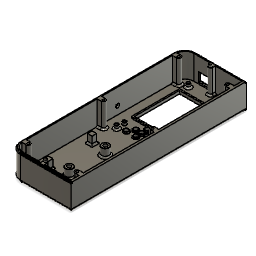
Front_panel_rev_C+ (Autodesk Fusion 360 design; units mm, degrees)
Autodesk Fusion 360 part; units mm, degrees
sketch "Sketch1" plane through (0, 0, 0) normal (0, 1, 0) x (1, 0, 0)
  line L0 (-20, 50) -> (62, 50)
  line L1 (62, 50) -> (62, -183)
  line L2 (62, -183) -> (-20, -183)
  line L3 (-20, -183) -> (-20, 50)
  dimension "d1" = 233
  dimension "d2" = 82
  dimension "d62" = 0
  dimension "d63" = 0
  dimension "d64" = 0
  dimension "d65" = 0
  constraint horizontal L0
  constraint vertical L1
  constraint horizontal L2
  constraint vertical L3
  measures "d1" distance of L0.start L2.end
  measures "d2" distance of L0.start L0.end
extrude "Extrude1" add sketch "Sketch1" along normal blind 35
fillet "Fillet1" radius 15 2 edges at (-20, 17.5, -50) (-20, 17.5, 183)
shell "Shell1" thickness 3 removed faces 1 at (34.6667, 35, 32.6667)
sketch "Sketch2" plane through (0, 35, 0) normal (0, 1, 0) x (-1, 0, 0)
  arc A0 (5, -47) -> (17, -35) centre (5, -35) ccw
  line L0 (5, -47) -> (-59, -47)
  line L1 (-59, -47) -> (-59, 180)
  line L2 (-59, 180) -> (5, 180)
  arc A1 (17, 168) -> (5, 180) centre (5, 168) ccw
  line L3 (17, 168) -> (17, -35)
  arc A2 (20, 168) -> (5, 183) centre (5, 168) ccw
  line L4 (5, 183) -> (-62, 183)
  line L5 (-62, 183) -> (-62, -50)
  line L6 (-62, -50) -> (5, -50)
  arc A3 (5, -50) -> (20, -35) centre (5, -35) ccw
  line L7 (20, -35) -> (20, 168)
  line L8 (-62, -48.5) -> (5, -48.5)
  arc A4 (5, -48.5) -> (18.5, -35) centre (5, -35) ccw
  line L9 (18.5, -35) -> (18.5, 168)
  arc A5 (18.5, 168) -> (5, 181.5) centre (5, 168) ccw
  line L10 (5, 181.5) -> (-62, 181.5)
  dimension "d7" = 1.5
extrude "Extrude2" cut sketch "Sketch2" against normal blind 1.6 contours A2 L4 L5 L6 A3 L7 L8 A4 L9 A5 L10
sketch "Sketch3" plane through (0, 3, 0) normal (0, 1, 0) x (-1, 0, 0)
  arc A0 (17, 168) -> (5, 180) centre (5, 168) ccw
  line L0 (5, 180) -> (-59, 180)
  line L1 (-59, 180) -> (-59, -47)
  line L2 (-59, -47) -> (5, -47)
  arc A1 (5, -47) -> (17, -35) centre (5, -35) ccw
  line L3 (17, -35) -> (17, 168)
  circle A2 centre (-21, 176) radius 2.5
  line L4 (-62, 181.5) -> (-62, -48.5)
  line L5 (-62, 183) -> (5, 183)
  circle A3 centre (-21, -43) radius 2.5
  line L6 (5, -50) -> (-62, -50)
  line L7 (20, 168) -> (20, -35) construction
  line L8 (-62, 66.5) -> (20, 66.5) construction
  circle A4 centre (11.5, 66.5) radius 3
  circle A5 centre (-53.5, 66.5) radius 3
  line L9 (-21, 230) -> (-21, -74.0636) construction
  line L10 (11.5, 191.1088) -> (11.5, -90) construction
  line L11 (-53.5, -65.1601) -> (-53.5, 224.5392) construction
  circle A6 centre (11.5, 166.5) radius 3
  circle A7 centre (-53.5, 166.5) radius 3
  circle A8 centre (11.5, -33.5) radius 3
  circle A9 centre (-53.5, -33.5) radius 3
  line L12 (-53.5, 169.5) -> (-59, 169.5)
  line L13 (-53.5, 163.5) -> (-59, 163.5)
  line L14 (11.5, 169.5) -> (16.9059, 169.5)
  line L15 (11.5, 163.5) -> (17, 163.5)
  line L16 (11.5, 63.5) -> (17, 63.5)
  line L17 (11.5, 69.5) -> (17, 69.5)
  line L18 (-53.5, 63.5) -> (-59, 63.5)
  line L19 (-53.5, 69.5) -> (-59, 69.5)
  line L20 (11.5, -36.5) -> (16.9059, -36.5)
  line L21 (11.5, -30.5) -> (17, -30.5)
  line L22 (-18.5, -43) -> (-18.5, -47)
  line L23 (-23.5, -43) -> (-23.5, -47)
  line L24 (-23.5, 176) -> (-23.5, 180)
  line L25 (-18.5, 176) -> (-18.5, 180)
  line L26 (-53.5, -30.5) -> (-59, -30.5)
  line L27 (-53.5, -36.5) -> (-59, -36.5)
  line L28 (-46.4, 61) -> (4.4, 61)
  line L29 (4.4, 61) -> (4.4, -39)
  line L30 (4.4, -39) -> (-46.4, -39)
  line L31 (-46.4, -39) -> (-46.4, 61)
  line L32 (-46.4, 61) -> (4.4, -39) construction
  line L33 (4.4, 61) -> (-46.4, -39) construction
  line L34 (-43.86, 58.625) -> (1.86, 58.625)
  line L35 (1.86, 58.625) -> (1.86, -36.625)
  line L36 (1.86, -36.625) -> (-43.86, -36.625)
  line L37 (-43.86, -36.625) -> (-43.86, 58.625)
  line L38 (-43.86, 58.625) -> (1.86, -36.625) construction
  line L39 (1.86, 58.625) -> (-43.86, -36.625) construction
  circle A10 centre (1.86, -36.625) radius 1.5
  circle A11 centre (-43.86, -36.625) radius 2.5
  circle A12 centre (-43.86, -36.625) radius 1.5
  circle A13 centre (1.86, -36.625) radius 2.5
  circle A14 centre (1.86, 58.625) radius 2.5
  circle A15 centre (1.86, 58.625) radius 1.5
  circle A16 centre (-43.86, 58.625) radius 2.5
  circle A17 centre (-43.86, 58.625) radius 1.5
  line L40 (-43.5, 149.6675) -> (1.5, 149.6675)
  line L41 (1.5, 149.6675) -> (1.5, 91.6675)
  line L42 (1.5, 91.6675) -> (-43.5, 91.6675)
  line L43 (-43.5, 91.6675) -> (-43.5, 149.6675)
  line L44 (-43.5, 149.6675) -> (1.5, 91.6675) construction
  line L45 (1.5, 149.6675) -> (-43.5, 91.6675) construction
  circle A18 centre (-21, 144.6675) radius 2.5
  circle A19 centre (-21, 96.6675) radius 2.5
  circle A20 centre (-21, 96.6675) radius 5
  circle A21 centre (-21, 144.6675) radius 5
  line L46 (-1.5, 94.6675) -> (4.5, 94.6675)
  line L47 (4.5, 94.6675) -> (4.5, 88.6675)
  line L48 (4.5, 88.6675) -> (-1.5, 88.6675)
  line L49 (-1.5, 88.6675) -> (-1.5, 94.6675)
  line L50 (-1.5, 94.6675) -> (4.5, 88.6675) construction
  line L51 (4.5, 94.6675) -> (-1.5, 88.6675) construction
  line L52 (-46.5, 94.6675) -> (-40.5, 94.6675)
  line L53 (-40.5, 94.6675) -> (-40.5, 88.6675)
  line L54 (-40.5, 88.6675) -> (-46.5, 88.6675)
  line L55 (-46.5, 88.6675) -> (-46.5, 94.6675)
  line L56 (-46.5, 94.6675) -> (-40.5, 88.6675) construction
  line L57 (-40.5, 94.6675) -> (-46.5, 88.6675) construction
  line L58 (-1.5, 152.6675) -> (4.5, 152.6675)
  line L59 (4.5, 152.6675) -> (4.5, 146.6675)
  line L60 (4.5, 146.6675) -> (-1.5, 146.6675)
  line L61 (-1.5, 146.6675) -> (-1.5, 152.6675)
  line L62 (-1.5, 152.6675) -> (4.5, 146.6675) construction
  line L63 (4.5, 152.6675) -> (-1.5, 146.6675) construction
  line L64 (-46.5, 152.6675) -> (-40.5, 152.6675)
  line L65 (-40.5, 152.6675) -> (-40.5, 146.6675)
  line L66 (-40.5, 146.6675) -> (-46.5, 146.6675)
  line L67 (-46.5, 146.6675) -> (-46.5, 152.6675)
  line L68 (-46.5, 152.6675) -> (-40.5, 146.6675) construction
  line L69 (-40.5, 152.6675) -> (-46.5, 146.6675) construction
  point P0 (-21, 11)
  point P1 (-21, 11)
  point P2 (-21, 120.6675)
  point P3 (1.5, 91.6675)
  point P4 (-43.5, 91.6675)
  point P5 (1.5, 149.6675)
  point P6 (-43.5, 149.6675)
  dimension "d10" = 41
  dimension "d11" = 7
  dimension "d12" = 41
  dimension "d13" = 7
  dimension "d14" = 5
  dimension "d15" = 5
  dimension "d16" = 6
  dimension "d17" = 6
  dimension "d18" = 32.5
  dimension "d19" = 32.5
  dimension "d20" = 6
  dimension "d21" = 6
  dimension "d22" = 6
  dimension "d23" = 6
  dimension "d24" = 100
  dimension "d25" = 100
  dimension "d26" = 100
  dimension "d27" = 100
  dimension "d42" = 41
  dimension "d43" = 100
  dimension "d44" = 50.8
  dimension "d45" = 61
  dimension "d46" = 45.72
  dimension "d47" = 95.25
  dimension "d48" = 3
  dimension "d49" = 5
  dimension "d50" = 3
  dimension "d51" = 5
  dimension "d52" = 5
  dimension "d53" = 3
  dimension "d54" = 5
  dimension "d55" = 3
  dimension "d86" = 58
  dimension "d87" = 45
  dimension "d88" = 5
  dimension "d89" = 5
  dimension "d90" = 24
  dimension "d91" = 24
  dimension "d92" = 10
  dimension "d93" = 10
  dimension "d94" = 6
  dimension "d95" = 6
  dimension "d96" = 6
  dimension "d97" = 6
  dimension "d98" = 6
  dimension "d99" = 6
  dimension "d100" = 6
  dimension "d101" = 6
  constraint midpoint L4 L8.start
  constraint midpoint L7 L8.end
  constraint coincident L8 A4.centre
  constraint coincident L8 A5.centre
  constraint perpendicular L8 L9
  constraint perpendicular L2 L10
  constraint perpendicular L5 L11
  constraint coincident L10 A6.centre
  constraint coincident L11 A7.centre
  constraint coincident L10 A8.centre
  constraint coincident L11 A9.centre
  constraint coincident A7 L12.start
  constraint coincident L11 L12.start
  constraint coincident L1 L12.end
  constraint coincident A7 L13.start
  constraint coincident L11 L13.start
  constraint coincident L1 L13.end
  constraint coincident A6 L14.start
  constraint coincident L10 L14.start
  constraint tangent A6 L14
  constraint coincident A6 L15.start
  constraint coincident L10 L15.start
  constraint tangent A6 L15
  constraint coincident L3 L15.end
  constraint coincident A0 L14.end
  constraint coincident A4 L16.start
  constraint coincident L10 L16.start
  constraint tangent A4 L16
  constraint perpendicular L3 L16
  constraint coincident A4 L17.start
  constraint coincident L10 L17.start
  constraint tangent A4 L17
  constraint coincident L3 L17.end
  constraint coincident L3 L16.end
  constraint coincident A5 L18.start
  constraint coincident L11 L18.start
  constraint tangent A5 L18
  constraint perpendicular L1 L18
  constraint coincident A5 L19.start
  constraint coincident L11 L19.start
  constraint tangent A5 L19
  constraint coincident L1 L18.end
  constraint coincident L1 L19.end
  constraint coincident A8 L20.start
  constraint coincident L10 L20.start
  constraint tangent A8 L20
  constraint coincident A8 L21.start
  constraint coincident L10 L21.start
  constraint tangent A8 L21
  constraint coincident L3 L21.end
  constraint coincident A1 L20.end
  constraint coincident A3 L22.start
  constraint perpendicular L2 L22
  constraint tangent A3 L22
  constraint coincident L2 L22.end
  constraint coincident A3 L23.start
  constraint perpendicular L2 L23
  constraint tangent A3 L23
  constraint coincident L2 L23.end
  constraint coincident A2 L24.start
  constraint perpendicular L0 L24
  constraint tangent A2 L24
  constraint coincident A2 L25.start
  constraint perpendicular L0 L25
  constraint tangent A2 L25
  constraint coincident L0 L25.end
  constraint coincident L0 L24.end
  constraint coincident A9 L26.start
  constraint perpendicular L11 L26
  constraint tangent A9 L26
  constraint coincident A9 L27.start
  constraint perpendicular L1 L27
  constraint tangent A9 L27
  constraint coincident L1 L27.end
  constraint coincident L1 L26.end
  constraint perpendicular L28 L29
  constraint parallel L28 L30
  constraint parallel L29 L31
  constraint horizontal L28
  constraint coincident L32 P1
  constraint coincident L33 P1
  constraint coincident L9 P1
  constraint perpendicular L34 L35
  constraint parallel L34 L36
  constraint parallel L35 L37
  constraint horizontal L34
  constraint coincident L38 P1
  constraint coincident L39 P1
  constraint coincident P1 P0
  constraint coincident L35.end L36.start
  constraint coincident L36.end L37.start
  constraint concentric A11 A12
  constraint concentric A10 A13
  constraint coincident L34.end L35.start
  constraint concentric A14 A15
  constraint coincident L34.start L37.end
  constraint concentric A16 A17
  constraint perpendicular L40 L41
  constraint parallel L40 L42
  constraint parallel L41 L43
  constraint horizontal L40
  constraint coincident L44 P2
  constraint coincident L45 P2
  constraint coincident L9 P2
  constraint coincident L9 A18.centre
  constraint coincident L9 A19.centre
  constraint concentric A19 A20
  constraint concentric A18 A21
  constraint perpendicular L46 L47
  constraint parallel L46 L48
  constraint parallel L47 L49
  constraint horizontal L46
  constraint coincident L50 P3
  constraint coincident L51 P3
  constraint coincident P3 L41.end
  constraint perpendicular L52 L53
  constraint parallel L52 L54
  constraint parallel L53 L55
  constraint horizontal L52
  constraint coincident L56 P4
  constraint coincident L57 P4
  constraint coincident P4 L42.end
  constraint perpendicular L58 L59
  constraint parallel L58 L60
  constraint parallel L59 L61
  constraint horizontal L58
  constraint coincident L62 P5
  constraint coincident L63 P5
  constraint coincident P5 L40.end
  constraint perpendicular L64 L65
  constraint parallel L64 L66
  constraint parallel L65 L67
  constraint horizontal L64
  constraint coincident L68 P6
  constraint coincident L69 P6
  constraint coincident P6 L40.start
  measures "d10" distance of A2.centre L4
  measures "d11" distance of A2.centre L5
  measures "d12" distance of L4 A3.centre
  measures "d13" distance of A3.centre L6
  measures "d14" diameter of A3
  measures "d15" diameter of A2
  measures "d16" diameter of A4
  measures "d17" diameter of A5
  measures "d18" distance of A5.centre L9
  measures "d19" distance of A4.centre L9
  measures "d20" diameter of A6
  measures "d21" diameter of A7
  measures "d22" diameter of A8
  measures "d23" diameter of A9
  measures "d24" distance of A4.centre A8.centre
  measures "d25" distance of A5.centre A9.centre
  measures "d26" distance of A4.centre A6.centre
  measures "d27" distance of A5.centre A7.centre
  measures "d42" distance of L4 L9
  measures "d43" distance of L28.end L29.end
  measures "d44" distance of L29.end L30.end
  measures "d45" distance of L6 P1
  measures "d46" distance of L35.end L36.end
  measures "d47" distance of L34.end L35.end
  measures "d48" diameter of A10
  measures "d49" diameter of A11
  measures "d50" diameter of A12
  measures "d51" diameter of A13
  measures "d52" diameter of A14
  measures "d53" diameter of A15
  measures "d54" diameter of A16
  measures "d55" diameter of A17
  measures "d86" distance of P5 P3
  measures "d87" distance of P3 P4
  measures "d88" diameter of A18
  measures "d89" diameter of A19
  measures "d90" distance of P2 A19.centre
  measures "d91" distance of P2 A18.centre
  measures "d92" diameter of A20
  measures "d93" diameter of A21
  measures "d94" distance of L47.end L48.end
  measures "d95" distance of L46.end L47.end
  measures "d96" distance of L53.end L54.end
  measures "d97" distance of L52.end L53.end
  measures "d98" distance of L58.end L59.end
  measures "d99" distance of L59.end L60.end
  measures "d100" distance of L64.end L65.end
  measures "d101" distance of L65.end L66.end
extrude "Extrude6" add sketch "Sketch3" along normal blind 5 contours L28 A16 | L28 L34 L37 A16 A17 | L34 L37 A16 A17 | L30 L36 L37 A11 A12 | L30 A11 | L28 A14 | L28 L34 L35 A14 A15 | L36 L37 A11 A12 | L34 L35 A14 A15 | L30 L35 L36 A10 A13 | L30 A13 | L35 L36 A10 A13
extrude "Extrude9" add sketch "Sketch3" along normal blind 11 contours L40 L43 L64 L65 L66 L67 | L40 L43 L65 L66 | A20 | A21 | L42 L43 L52 L53 | L42 L43 L52 L53 L54 L55 | L40 L41 L58 L59 L60 L61 | L40 L41 L60 L61 | L41 L42 L46 L47 L48 L49 | L41 L42 L46 L49
extrude "Extrude3" add sketch "Sketch3" along normal up to surface (32 mm away) contours A0 L3 A6 L14 L15 | A6 | L3 A4 L16 L17 | L0 A2 L24 L25 | A4 | A2 | A1 L3 A8 L20 L21 | A8 | L1 A7 L12 L13 | A7 | L1 A5 L18 L19 | L2 A3 L22 L23 | A5 | A3 | L1 A9 L26 L27 | A9
fillet "Fillet3" radius 2 46 edges at (0.4708, 3, 59.529) (25.6616, 3, 98.4755) (46.1908, 3, 59.529) (0.4708, 3, -35.721) (-14.2029, 3, -36.5) (-8.5, 3, -33.5) (-14.25, 3, -30.5) (23.5, 3, -45) (21, 3, -40.5) (18.5, 3, -45) (46.1908, 3, -35.721) (56.25, 3, -30.5) (50.5, 3, -33.5) (56.25, 3, -36.5) (56.25, 3, 69.5) (50.5, 3, 66.5) (56.25, 3, 63.5) (56.25, 3, 169.5) (50.5, 3, 166.5) (56.25, 3, 163.5) (18.5, 3, 178) (21, 3, 173.5) (23.5, 3, 178) (25.6616, 3, 146.4755) (-14.25, 3, 163.5) (-8.5, 3, 166.5) (-14.2029, 3, 169.5) (-1.5, 3, 146.6675) (1.5, 3, 149.6675) (-4.5, 3, 149.6675) (-1.5, 3, 152.6675) (-1.5, 3, 88.6675) (-1.5, 3, 94.6675) (-4.5, 3, 91.6675) (43.5, 3, 146.6675) (40.5, 3, 149.6675) (43.5, 3, 152.6675) (46.5, 3, 149.6675) (43.5, 3, 88.6675) (40.5, 3, 91.6675) (43.5, 3, 94.6675) (46.5, 3, 91.6675) (1.5, 3, 91.6675) (-14.25, 3, 63.5) (-8.5, 3, 66.5) (-14.25, 3, 69.5)
sketch "Sketch4" plane through (0, 35, 0) normal (0, 1, 0) x (-1, 0, 0)
  line L0 (5, 181.5) -> (-62, 181.5)
  line L1 (-62, 181.5) -> (-62, -48.5)
  line L2 (-62, -48.5) -> (5, -48.5)
  arc A0 (5, -48.5) -> (18.5, -35) centre (5, -35) ccw
  line L3 (18.5, -35) -> (18.5, 168)
  arc A1 (18.5, 168) -> (5, 181.5) centre (5, 168) ccw
  arc A2 (5, -47) -> (16.9059, -36.5) centre (5, -35) ccw
  line L4 (5, -47) -> (-18.5, -47)
  line L5 (-18.5, -47) -> (-18.5, -43)
  arc A3 (-18.5, -43) -> (-23.5, -43) centre (-21, -43) ccw
  line L6 (-23.5, -43) -> (-23.5, -47)
  line L7 (-23.5, -47) -> (-59, -47)
  line L8 (-59, -47) -> (-59, -36.5)
  line L9 (-59, -36.5) -> (-53.5, -36.5)
  arc A4 (-53.5, -36.5) -> (-53.5, -30.5) centre (-53.5, -33.5) ccw
  line L10 (-53.5, -30.5) -> (-59, -30.5)
  line L11 (-59, -30.5) -> (-59, 63.5)
  line L12 (-59, 63.5) -> (-53.5, 63.5)
  arc A5 (-53.5, 63.5) -> (-53.5, 69.5) centre (-53.5, 66.5) ccw
  line L13 (-53.5, 69.5) -> (-59, 69.5)
  line L14 (-59, 69.5) -> (-59, 163.5)
  line L15 (-59, 163.5) -> (-53.5, 163.5)
  arc A6 (-53.5, 163.5) -> (-53.5, 169.5) centre (-53.5, 166.5) ccw
  line L16 (-53.5, 169.5) -> (-59, 169.5)
  line L17 (-59, 169.5) -> (-59, 180)
  line L18 (-59, 180) -> (-23.5, 180)
  line L19 (-23.5, 180) -> (-23.5, 176)
  arc A7 (-23.5, 176) -> (-18.5, 176) centre (-21, 176) ccw
  line L20 (-18.5, 176) -> (-18.5, 180)
  line L21 (-18.5, 180) -> (5, 180)
  arc A8 (16.9059, 169.5) -> (5, 180) centre (5, 168) ccw
  line L22 (16.9059, 169.5) -> (11.5, 169.5)
  arc A9 (11.5, 169.5) -> (11.5, 163.5) centre (11.5, 166.5) ccw
  line L23 (11.5, 163.5) -> (17, 163.5)
  line L24 (17, 163.5) -> (17, 69.5)
  line L25 (17, 69.5) -> (11.5, 69.5)
  arc A10 (11.5, 69.5) -> (11.5, 63.5) centre (11.5, 66.5) ccw
  line L26 (11.5, 63.5) -> (17, 63.5)
  line L27 (17, 63.5) -> (17, -30.5)
  line L28 (17, -30.5) -> (11.5, -30.5)
  arc A11 (11.5, -30.5) -> (11.5, -36.5) centre (11.5, -33.5) ccw
  line L29 (11.5, -36.5) -> (16.9059, -36.5)
  circle A12 centre (-21, -43) radius 1.75
  circle A13 centre (-21, 176) radius 1.75
  dimension "d30" = 3.5
  dimension "d31" = 3.5
  constraint concentric A3 A12
  constraint concentric A7 A13
  measures "d30" diameter of A12
  measures "d31" diameter of A13
extrude "Extrude4" add sketch "Sketch4" along normal blind 3 contours A12 | A13
sketch "Sketch5" plane through (0, 35, 0) normal (0, 1, 0) x (-1, 0, 0)
  circle A0 centre (-21, -43) radius 1.75
  circle A1 centre (-21, 176) radius 1.75
  line L0 (5, 181.5) -> (-62, 181.5)
  line L1 (-62, 181.5) -> (-62, -48.5)
  line L2 (-62, -48.5) -> (5, -48.5)
  arc A2 (5, -48.5) -> (18.5, -35) centre (5, -35) ccw
  line L3 (18.5, -35) -> (18.5, 168)
  arc A3 (18.5, 168) -> (5, 181.5) centre (5, 168) ccw
  arc A4 (5, -47) -> (16.9059, -36.5) centre (5, -35) ccw
  line L4 (5, -47) -> (-18.5, -47)
  line L5 (-18.5, -47) -> (-18.5, -43)
  arc A5 (-18.5, -43) -> (-23.5, -43) centre (-21, -43) ccw
  line L6 (-23.5, -43) -> (-23.5, -47)
  line L7 (-23.5, -47) -> (-59, -47)
  line L8 (-59, -47) -> (-59, -36.5)
  line L9 (-59, -36.5) -> (-53.5, -36.5)
  arc A6 (-53.5, -36.5) -> (-53.5, -30.5) centre (-53.5, -33.5) ccw
  line L10 (-53.5, -30.5) -> (-59, -30.5)
  line L11 (-59, -30.5) -> (-59, 63.5)
  line L12 (-59, 63.5) -> (-53.5, 63.5)
  arc A7 (-53.5, 63.5) -> (-53.5, 69.5) centre (-53.5, 66.5) ccw
  line L13 (-53.5, 69.5) -> (-59, 69.5)
  line L14 (-59, 69.5) -> (-59, 163.5)
  line L15 (-59, 163.5) -> (-53.5, 163.5)
  arc A8 (-53.5, 163.5) -> (-53.5, 169.5) centre (-53.5, 166.5) ccw
  line L16 (-53.5, 169.5) -> (-59, 169.5)
  line L17 (-59, 169.5) -> (-59, 180)
  line L18 (-59, 180) -> (-23.5, 180)
  line L19 (-23.5, 180) -> (-23.5, 176)
  arc A9 (-23.5, 176) -> (-18.5, 176) centre (-21, 176) ccw
  line L20 (-18.5, 176) -> (-18.5, 180)
  line L21 (-18.5, 180) -> (5, 180)
  arc A10 (16.9059, 169.5) -> (5, 180) centre (5, 168) ccw
  line L22 (16.9059, 169.5) -> (11.5, 169.5)
  arc A11 (11.5, 169.5) -> (11.5, 163.5) centre (11.5, 166.5) ccw
  line L23 (11.5, 163.5) -> (17, 163.5)
  line L24 (17, 163.5) -> (17, 69.5)
  line L25 (17, 69.5) -> (11.5, 69.5)
  arc A12 (11.5, 69.5) -> (11.5, 63.5) centre (11.5, 66.5) ccw
  line L26 (11.5, 63.5) -> (17, 63.5)
  line L27 (17, 63.5) -> (17, -30.5)
  line L28 (17, -30.5) -> (11.5, -30.5)
  arc A13 (11.5, -30.5) -> (11.5, -36.5) centre (11.5, -33.5) ccw
  line L29 (11.5, -36.5) -> (16.9059, -36.5)
  circle A14 centre (11.5, 66.5) radius 1.5
  circle A15 centre (-53.5, 66.5) radius 1.5
  circle A16 centre (11.5, 166.5) radius 1.5
  circle A17 centre (-53.5, 166.5) radius 1.5
  circle A18 centre (11.5, -33.5) radius 1.5
  circle A19 centre (-53.5, -33.5) radius 1.5
  dimension "d34" = 3
  dimension "d35" = 3
  dimension "d36" = 3
  dimension "d37" = 3
  dimension "d38" = 3
  dimension "d39" = 3
  constraint concentric A12 A14
  constraint concentric A7 A15
  constraint concentric A11 A16
  constraint concentric A8 A17
  constraint concentric A13 A18
  constraint concentric A6 A19
  measures "d34" diameter of A14
  measures "d35" diameter of A15
  measures "d36" diameter of A16
  measures "d37" diameter of A17
  measures "d38" diameter of A18
  measures "d39" diameter of A19
extrude "Extrude5" cut sketch "Sketch5" against normal blind 15 contours A14 | A15 | A16 | A17 | A18 | A19
sketch "Sketch6" plane through (0, 0, 0) normal (0, -1, 0) x (1, 0, 0)
  line L0 (-4, -32.555) -> (46, -32.555)
  line L1 (46, -32.555) -> (46, 36.645)
  line L2 (46, 36.645) -> (-4, 36.645)
  line L3 (-4, 36.645) -> (-4, -32.555)
  line L4 (59, -47) -> (25.5, -47)
  arc A0 (-16.4782, -38.5) -> (-5, -47) centre (-5, -35) ccw
  line L5 (-17, 71.5) -> (-17, 161.5)
  line L6 (-4, -32.555) -> (46, 36.645) construction
  line L7 (46, -32.555) -> (-4, 36.645) construction
  line L8 (44, 32.045) -> (-2, -27.955) construction
  line L9 (-2, 32.045) -> (44, -27.955) construction
  circle A1 centre (13.38, 48.465) radius 0.9492
  circle A2 centre (21, 48.465) radius 0.9492
  circle A3 centre (21, 56.085) radius 0.9492
  circle A4 centre (28.62, 48.465) radius 0.9492
  circle A5 centre (21, 40.845) radius 0.9492
  line L10 (-11.5, 71.5) -> (-17, 71.5)
  line L11 (-17, 161.5) -> (-11.5, 161.5)
  arc A6 (-11.5, 161.5) -> (-11.5, 171.5) centre (-11.5, 166.5) ccw
  line L12 (-11.5, 171.5) -> (-16.4782, 171.5)
  line L13 (16.5, 180) -> (16.5, 176)
  arc A7 (16.5, 176) -> (25.5, 176) centre (21, 176) ccw
  line L14 (25.5, 176) -> (25.5, 180)
  line L15 (59, 171.5) -> (53.5, 171.5)
  arc A8 (53.5, 171.5) -> (53.5, 161.5) centre (53.5, 166.5) ccw
  line L16 (53.5, 161.5) -> (59, 161.5)
  line L17 (59, 161.5) -> (59, 71.5)
  line L18 (59, 71.5) -> (53.5, 71.5)
  arc A9 (53.5, 71.5) -> (53.5, 61.5) centre (53.5, 66.5) ccw
  line L19 (53.5, 61.5) -> (59, 61.5)
  line L20 (59, 61.5) -> (59, -28.5)
  line L21 (59, -28.5) -> (53.5, -28.5)
  arc A10 (53.5, -28.5) -> (53.5, -38.5) centre (53.5, -33.5) ccw
  line L22 (53.5, -38.5) -> (59, -38.5)
  line L23 (59, -38.5) -> (59, -47)
  line L24 (25.5, -47) -> (25.5, -43)
  arc A11 (25.5, -43) -> (16.5, -43) centre (21, -43) ccw
  line L25 (16.5, -43) -> (16.5, -47)
  line L26 (-16.4782, -38.5) -> (-11.5, -38.5)
  arc A12 (-11.5, -38.5) -> (-11.5, -28.5) centre (-11.5, -33.5) ccw
  line L27 (-11.5, -28.5) -> (-17, -28.5)
  line L28 (-17, -28.5) -> (-17, 61.5)
  line L29 (-17, 61.5) -> (-11.5, 61.5)
  arc A13 (-11.5, 61.5) -> (-11.5, 71.5) centre (-11.5, 66.5) ccw
  line L30 (38.5, 154.6675) -> (38.5, 144.6675)
  line L31 (38.5, 144.6675) -> (48.5, 144.6675)
  line L32 (48.5, 144.6675) -> (48.5, 154.6675)
  line L33 (48.5, 154.6675) -> (38.5, 154.6675)
  line L34 (-6.5, 154.6675) -> (-6.5, 144.6675)
  line L35 (-6.5, 144.6675) -> (3.5, 144.6675)
  line L36 (3.5, 144.6675) -> (3.5, 154.6675)
  line L37 (3.5, 154.6675) -> (-6.5, 154.6675)
  circle A14 centre (43.86, -36.625) radius 4.5
  circle A15 centre (43.86, 58.625) radius 4.5
  circle A16 centre (-1.86, 58.625) radius 4.5
  circle A17 centre (21, 96.6675) radius 7
  circle A18 centre (-1.86, -36.625) radius 4.5
  circle A19 centre (21, 144.6675) radius 7
  line L38 (-6.5, 96.6675) -> (-6.5, 86.6675)
  line L39 (-6.5, 86.6675) -> (3.5, 86.6675)
  line L40 (3.5, 86.6675) -> (3.5, 96.6675)
  line L41 (3.5, 96.6675) -> (-6.5, 96.6675)
  line L42 (38.5, 96.6675) -> (38.5, 86.6675)
  line L43 (38.5, 86.6675) -> (48.5, 86.6675)
  line L44 (48.5, 86.6675) -> (48.5, 96.6675)
  line L45 (48.5, 96.6675) -> (38.5, 96.6675)
  arc A20 (-5, 183) -> (-20, 168) centre (-5, 168) ccw
  line L46 (-20, 168) -> (-20, -35)
  arc A21 (-20, -35) -> (-5, -50) centre (-5, -35) ccw
  line L47 (-5, -50) -> (62, -50)
  line L48 (62, -50) -> (62, 183)
  line L49 (62, 183) -> (-5, 183)
  circle A22 centre (33.7, 56.085) radius 0.9492
  circle A23 centre (8.3, 56.085) radius 0.9492
  line L50 (-2, 35.045) -> (44, 35.045)
  line L51 (44, 35.045) -> (44, -24.955)
  line L52 (44, -24.955) -> (-2, -24.955)
  line L53 (-2, -24.955) -> (-2, 35.045)
  line L54 (-2, 35.045) -> (44, -24.955) construction
  line L55 (44, 35.045) -> (-2, -24.955) construction
  point P0 (21, 2.045)
  point P1 (21, 5.045)
  dimension "d80" = 46
  dimension "d81" = 60
  dimension "d138" = 12.7
  dimension "d139" = 12.7
  dimension "d146" = 46
  dimension "d147" = 60
  dimension "d148" = 3
  constraint coincident L0.start L3.end
  constraint coincident L1.end L2.start
  constraint coincident L0.end L1.start
  constraint coincident L2.end L3.start
  constraint coincident L8 P0
  constraint coincident L9 P0
  constraint midpoint L6 P0
  constraint equal A3 A23
  constraint equal A3 A22
  constraint perpendicular L50 L51
  constraint parallel L50 L52
  constraint parallel L51 L53
  constraint horizontal L50
  constraint coincident L54 P1
  constraint coincident L55 P1
  measures "d80" distance of L8.end L9.end
  measures "d81" distance of L9.start L8.end
  measures "d138" distance of A3.centre A22.centre
  measures "d139" distance of A3.centre A23.centre
  measures "d146" distance of L51.end L52.end
  measures "d147" distance of L50.end L51.end
  measures "d148" distance of P0 P1
extrude "Extrude7" cut sketch "Sketch6" against normal blind 5 contours A1 | A2 | A3 | A4 | A5 | A22 | A23 | L50 L51 L52 L53
sketch "Sketch7" plane through (0, 3, 0) normal (0, 1, 0) x (-1, 0, 0)
  circle A0 centre (-21, 48.465) radius 0.9492
  circle A1 centre (-13.38, 48.465) radius 0.9492
  circle A2 centre (-28.62, 48.465) radius 0.9492
  circle A3 centre (-21, 40.845) radius 0.9492
  circle A4 centre (-21, 56.085) radius 0.9492
  line L0 (-59, 180) -> (-59, 171.5)
  line L1 (-59, -47) -> (-25.5, -47)
  line L2 (-16.5, -47) -> (5, -47)
  arc A5 (5, -47) -> (16.4782, -38.5) centre (5, -35) ccw
  line L3 (17, 71.5) -> (17, 161.5)
  arc A6 (16.4782, 171.5) -> (5, 180) centre (5, 168) ccw
  line L4 (5, 180) -> (-16.5, 180)
  line L5 (-25.5, 180) -> (-59, 180)
  line L6 (11.5, 71.5) -> (17, 71.5)
  line L7 (17, 161.5) -> (11.5, 161.5)
  arc A7 (11.5, 171.5) -> (11.5, 161.5) centre (11.5, 166.5) ccw
  line L8 (11.5, 171.5) -> (16.4782, 171.5)
  line L9 (-16.5, 180) -> (-16.5, 176)
  arc A8 (-25.5, 176) -> (-16.5, 176) centre (-21, 176) ccw
  line L10 (-25.5, 176) -> (-25.5, 180)
  line L11 (-59, 171.5) -> (-53.5, 171.5)
  arc A9 (-53.5, 161.5) -> (-53.5, 171.5) centre (-53.5, 166.5) ccw
  line L12 (-53.5, 161.5) -> (-59, 161.5)
  line L13 (-59, 161.5) -> (-59, 71.5)
  line L14 (-59, 71.5) -> (-53.5, 71.5)
  arc A10 (-53.5, 61.5) -> (-53.5, 71.5) centre (-53.5, 66.5) ccw
  line L15 (-53.5, 61.5) -> (-59, 61.5)
  line L16 (-59, 61.5) -> (-59, -28.5)
  line L17 (-59, -28.5) -> (-53.5, -28.5)
  arc A11 (-53.5, -38.5) -> (-53.5, -28.5) centre (-53.5, -33.5) ccw
  line L18 (-53.5, -38.5) -> (-59, -38.5)
  line L19 (-59, -38.5) -> (-59, -47)
  line L20 (-25.5, -47) -> (-25.5, -43)
  arc A12 (-16.5, -43) -> (-25.5, -43) centre (-21, -43) ccw
  line L21 (-16.5, -43) -> (-16.5, -47)
  line L22 (16.4782, -38.5) -> (11.5, -38.5)
  arc A13 (11.5, -28.5) -> (11.5, -38.5) centre (11.5, -33.5) ccw
  line L23 (11.5, -28.5) -> (17, -28.5)
  line L24 (17, -28.5) -> (17, 61.5)
  line L25 (17, 61.5) -> (11.5, 61.5)
  arc A14 (11.5, 71.5) -> (11.5, 61.5) centre (11.5, 66.5) ccw
  line L26 (-38.5, 154.6675) -> (-38.5, 144.6675)
  line L27 (-38.5, 144.6675) -> (-48.5, 144.6675)
  line L28 (-48.5, 144.6675) -> (-48.5, 154.6675)
  line L29 (-48.5, 154.6675) -> (-38.5, 154.6675)
  line L30 (6.5, 154.6675) -> (6.5, 144.6675)
  line L31 (6.5, 144.6675) -> (-3.5, 144.6675)
  line L32 (-3.5, 144.6675) -> (-3.5, 154.6675)
  line L33 (-3.5, 154.6675) -> (6.5, 154.6675)
  circle A15 centre (-43.86, 58.625) radius 4.5
  circle A16 centre (1.86, 58.625) radius 4.5
  circle A17 centre (-21, 96.6675) radius 7
  circle A18 centre (-21, 144.6675) radius 7
  line L34 (6.5, 96.6675) -> (6.5, 86.6675)
  line L35 (6.5, 86.6675) -> (-3.5, 86.6675)
  line L36 (-3.5, 86.6675) -> (-3.5, 96.6675)
  line L37 (-3.5, 96.6675) -> (6.5, 96.6675)
  line L38 (-38.5, 96.6675) -> (-38.5, 86.6675)
  line L39 (-38.5, 86.6675) -> (-48.5, 86.6675)
  line L40 (-48.5, 86.6675) -> (-48.5, 96.6675)
  line L41 (-48.5, 96.6675) -> (-38.5, 96.6675)
  circle A19 centre (1.8403, 48.465) radius 1.5
  circle A20 centre (-43.86, -36.625) radius 4.5
  circle A21 centre (1.86, -36.625) radius 4.5
  circle A22 centre (-33.7, 56.085) radius 0.9492
  circle A23 centre (-8.3, 56.085) radius 0.9492
  line L42 (-44, -24.955) -> (-44, 35.045)
  line L43 (-44, 35.045) -> (2, 35.045)
  line L44 (2, 35.045) -> (2, -24.955)
  line L45 (2, -24.955) -> (-44, -24.955)
  line L46 (-46, 37.045) -> (4, 37.045)
  line L47 (4, 37.045) -> (4, -26.955)
  line L48 (4, -26.955) -> (-46, -26.955)
  line L49 (-46, -26.955) -> (-46, 37.045)
  dimension "d119" = 3
  dimension "d150" = -2
  measures "d119" diameter of A19
extrude "Extrude12" cut sketch "Sketch7" against normal up to surface (3 mm away) contours A19
extrude "Extrude8" add sketch "Sketch7" along normal blind 2 contours L46 L47 L48 L49
move_face "OffsetFaces1" offset -1.5 7 faces at (14.1366, 2, 49.0381) (21.7566, 2, 41.4181) (21.7566, 2, 49.0381) (29.3766, 2, 49.0381) (21.7566, 2, 56.6581) (9.0566, 2, 56.6581) (34.4566, 2, 56.6581)
sketch "Sketch9" plane through (0, 3, 0) normal (0, 1, 0) x (-1, 0, 0)
  circle A0 centre (-21, 48.465) radius 2.4492
  circle A1 centre (-13.38, 48.465) radius 2.4492
  circle A2 centre (-28.62, 48.465) radius 2.4492
  circle A3 centre (-21, 40.845) radius 2.4492
  circle A4 centre (-21, 56.085) radius 2.4492
  line L0 (11.5, 71.5) -> (17, 71.5)
  line L1 (17, 71.5) -> (17, 161.5)
  line L2 (17, 161.5) -> (11.5, 161.5)
  arc A5 (11.5, 171.5) -> (11.5, 161.5) centre (11.5, 166.5) ccw
  line L3 (11.5, 171.5) -> (16.4782, 171.5)
  arc A6 (16.4782, 171.5) -> (5, 180) centre (5, 168) ccw
  line L4 (5, 180) -> (-16.5, 180)
  line L5 (-16.5, 180) -> (-16.5, 176)
  arc A7 (-25.5, 176) -> (-16.5, 176) centre (-21, 176) ccw
  line L6 (-25.5, 176) -> (-25.5, 180)
  line L7 (-25.5, 180) -> (-59, 180)
  line L8 (-59, 180) -> (-59, 171.5)
  line L9 (-59, 171.5) -> (-53.5, 171.5)
  arc A8 (-53.5, 161.5) -> (-53.5, 171.5) centre (-53.5, 166.5) ccw
  line L10 (-53.5, 161.5) -> (-59, 161.5)
  line L11 (-59, 161.5) -> (-59, 71.5)
  line L12 (-59, 71.5) -> (-53.5, 71.5)
  arc A9 (-53.5, 61.5) -> (-53.5, 71.5) centre (-53.5, 66.5) ccw
  line L13 (-53.5, 61.5) -> (-59, 61.5)
  line L14 (-59, 61.5) -> (-59, -28.5)
  line L15 (-59, -28.5) -> (-53.5, -28.5)
  arc A10 (-53.5, -38.5) -> (-53.5, -28.5) centre (-53.5, -33.5) ccw
  line L16 (-53.5, -38.5) -> (-59, -38.5)
  line L17 (-59, -38.5) -> (-59, -47)
  line L18 (-59, -47) -> (-25.5, -47)
  line L19 (-25.5, -47) -> (-25.5, -43)
  arc A11 (-16.5, -43) -> (-25.5, -43) centre (-21, -43) ccw
  line L20 (-16.5, -43) -> (-16.5, -47)
  line L21 (-16.5, -47) -> (5, -47)
  arc A12 (5, -47) -> (16.4782, -38.5) centre (5, -35) ccw
  line L22 (16.4782, -38.5) -> (11.5, -38.5)
  arc A13 (11.5, -28.5) -> (11.5, -38.5) centre (11.5, -33.5) ccw
  line L23 (11.5, -28.5) -> (17, -28.5)
  line L24 (17, -28.5) -> (17, 61.5)
  line L25 (17, 61.5) -> (11.5, 61.5)
  arc A14 (11.5, 71.5) -> (11.5, 61.5) centre (11.5, 66.5) ccw
  line L26 (-38.5, 154.6675) -> (-38.5, 144.6675)
  line L27 (-38.5, 144.6675) -> (-48.5, 144.6675)
  line L28 (-48.5, 144.6675) -> (-48.5, 154.6675)
  line L29 (-48.5, 154.6675) -> (-38.5, 154.6675)
  line L30 (6.5, 154.6675) -> (6.5, 144.6675)
  line L31 (6.5, 144.6675) -> (-3.5, 144.6675)
  line L32 (-3.5, 144.6675) -> (-3.5, 154.6675)
  line L33 (-3.5, 154.6675) -> (6.5, 154.6675)
  circle A15 centre (-43.86, 58.625) radius 4.5
  circle A16 centre (1.86, 58.625) radius 4.5
  circle A17 centre (-21, 96.6675) radius 7
  circle A18 centre (-21, 144.6675) radius 7
  line L34 (6.5, 96.6675) -> (6.5, 86.6675)
  line L35 (6.5, 86.6675) -> (-3.5, 86.6675)
  line L36 (-3.5, 86.6675) -> (-3.5, 96.6675)
  line L37 (-3.5, 96.6675) -> (6.5, 96.6675)
  line L38 (-38.5, 96.6675) -> (-38.5, 86.6675)
  line L39 (-38.5, 86.6675) -> (-48.5, 86.6675)
  line L40 (-48.5, 86.6675) -> (-48.5, 96.6675)
  line L41 (-48.5, 96.6675) -> (-38.5, 96.6675)
  circle A19 centre (-21, 48.465) radius 3.4492
  circle A20 centre (-21, 40.845) radius 3.4492
  circle A21 centre (-13.38, 48.465) radius 3.4492
  circle A22 centre (-28.62, 48.465) radius 3.4492
  circle A23 centre (-21, 56.085) radius 3.4492
  circle A24 centre (1.8403, 48.465) radius 1.5
  circle A25 centre (1.8403, 48.465) radius 2.5
  circle A26 centre (-43.86, -36.625) radius 4.5
  circle A27 centre (1.86, -36.625) radius 4.5
  circle A28 centre (-33.7, 56.085) radius 2.4492
  circle A29 centre (-8.3, 56.085) radius 2.4492
  circle A30 centre (-8.3, 56.085) radius 3.4492
  circle A31 centre (-33.7, 56.085) radius 3.4492
  line L42 (-46, -26.955) -> (-46, 37.045)
  line L43 (-46, 37.045) -> (4, 37.045)
  line L44 (4, 37.045) -> (4, -26.955)
  line L45 (4, -26.955) -> (-46, -26.955)
  dimension "d111" = 1
  dimension "d112" = 1
  dimension "d113" = 1
  dimension "d114" = 1
  dimension "d115" = 1
  dimension "d122" = 1
  dimension "d140" = 1
  dimension "d141" = 1
extrude "Extrude13" add sketch "Sketch9" along normal blind 3.5 contours A25
extrude "Extrude11" add sketch "Sketch9" along normal blind 2 contours A19 | A20 | A21 | A22 | A23 | A30 | A31
fillet "Fillet5" chord length 0.5 20 edges at (24.2158, 3, 49.7123) (24.2158, 3, 57.3323) (31.8358, 3, 49.7123) (24.2158, 3, 42.0923) (16.5958, 3, 49.7123) (24.2158, 5, 47.2177) (24.2158, 5, 54.8377) (31.8358, 5, 47.2177) (24.2158, 5, 39.5977) (16.5958, 5, 47.2177) (0.4708, 8, 57.721) (46.1908, 8, 57.721) (25.6616, 14, 94.8594) (25.6616, 14, 142.8594) (0.4905, 6.5, 47.561) (0.4905, 3, 49.369) (0.4708, 8, -37.529) (46.1908, 8, -37.529) (11.5158, 3, 57.3323) (36.9158, 3, 57.3323)
fillet "Fillet2" radius 4 6 edges at (62, 0, 66.5) (28.5, 0, 183) (-15.6066, 0, 178.6066) (-20, 0, 66.5) (-15.6066, 0, -45.6066) (28.5, 0, -50)
sketch "Sketch8" plane through (0, 0, -50) normal (0, 0, -1) x (-1, 0, 0)
  line L0 (-62, 4) -> (5, 4)
  line L1 (5, 4) -> (5, 33.4)
  line L2 (5, 33.4) -> (-62, 33.4)
  line L3 (-62, 33.4) -> (-62, 4)
  line L4 (-2.055, 6.0851) -> (-17.055, 6.0851)
  line L5 (-17.055, 6.0851) -> (-17.055, 16.0851)
  line L6 (-17.055, 16.0851) -> (-2.055, 16.0851)
  line L7 (-2.055, 16.0851) -> (-2.055, 6.0851)
  line L8 (-2.055, 6.0851) -> (-17.055, 16.0851) construction
  line L9 (-17.055, 6.0851) -> (-2.055, 16.0851) construction
  line L10 (-9.76, 11.0851) -> (-9.35, 11.0851)
  line L11 (-62, 4) -> (5, 4)
  line L12 (5, 4) -> (5, 33.4)
  line L13 (5, 33.4) -> (-62, 33.4)
  line L14 (-62, 33.4) -> (-62, 4)
  point P0 (-9.555, 11.0851)
  dimension "d106" = 15
  dimension "d107" = 10
  constraint perpendicular L4 L5
  constraint parallel L4 L6
  constraint parallel L5 L7
  constraint horizontal L4
  constraint coincident L8 P0
  constraint coincident L9 P0
  constraint midpoint P0 L10
  measures "d106" distance of L5.end L6.end
  measures "d107" distance of L4.end L5.end
extrude "Extrude10" cut sketch "Sketch8" against normal up to surface (3 mm away) contours L4 L5 L6 L7
fillet "Fillet4" radius 1 18 edges at (9.555, 6.0851, -50) (2.055, 11.0851, -50) (9.555, 16.0851, -50) (17.055, 11.0851, -50) (9.555, 16.0851, -47) (2.055, 11.0851, -47) (9.555, 6.0851, -47) (17.055, 11.0851, -47) (18.7165, 0, 56.9707) (11.0965, 0, 49.3507) (18.7165, 0, 49.3507) (18.7165, 0, 41.7307) (26.3365, 0, 49.3507) (-0.4418, 0, 47.9226) (-2, 0, 5.045) (21, 0, 35.045) (44, 0, 5.045) (21, 0, -24.955)
sketch "Sketch10" plane through (-17, 0, 0) normal (1, 0, 0) x (0, 0, -1)
  arc A0 (-63.5, 5) -> (-61.5, 3) centre (-61.5, 5) ccw
  line L0 (-61.5, 3) -> (28.5, 3)
  arc A1 (28.5, 3) -> (30.5, 5) centre (28.5, 5) ccw
  line L1 (30.5, 5) -> (30.5, 35)
  line L2 (30.5, 35) -> (-63.5, 35)
  line L3 (-63.5, 35) -> (-63.5, 5)
  circle A2 centre (-42.242, 13.5744) radius 1.6294
  circle A3 centre (-42.242, 13.5744) radius 2.6294
  dimension "d142" = 1
extrude "Extrude14" cut sketch "Sketch10" against normal up to surface (3 mm away) contours A2 | A3
fillet "Fillet6" radius 1 1 edges at (-20, 12.6236, 44.6935)
equation "d18 = ( 65 / 2 ) * 1 mm"
equation "d19 = ( 65 / 2 ) * 1 mm"
equation "d25 = d24"
equation "d26 = d24"
equation "d27 = d24"
equation "d90 = ( 48 / 2 ) * 1 mm"
equation "d91 = ( 48 / 2 ) * 1 mm"
equation "d139 = d138"
